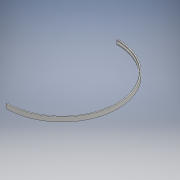
# Autodesk Inventor part: 異形橡膠圈-半圓
Saved by Autodesk Inventor 2018 (Build 220112000, 112)
## iProperties
Created: 2026-01-20
Part Number: 異形橡膠圈-半圓
Material: 一般
Document SubType Name: Modeling
Designer: User
Density: 1 g/cm^3
Appearance: 預設
Author: User
Autodesk Inventor part; units mm, degrees
ref_plane "YZ Plane" through (0, 0, 0) normal (1, 0, 0) x (0, 1, 0)
ref_plane "XZ Plane" through (0, 0, 0) normal (0, 1, 0) x (-1, 0, 0)
ref_plane "XY Plane" through (0, 0, 0) normal (0, 0, 1) x (1, 0, 0)
sketch "草圖1" plane through (0, 0, 0) normal (1, 0, 0) x (0, 1, 0)
  line L0 (-312, 12.65) -> (-317, 12.65)
  line L1 (-317, 12.65) -> (-317, -12.65)
  line L2 (-317, -12.65) -> (-312, -12.65)
  line L3 (-308, -12.65) -> (-308, 12.65) construction
  arc A0 (-310.3276, -7.5781) -> (-310.3276, 7.5781) centre (-321.5, 0) ccw
  line L4 (-310.5, -8.1394) -> (-310.5, -11.15)
  line L5 (-310.5, 8.1394) -> (-310.5, 11.15)
  arc A1 (-310.3276, -7.5781) -> (-310.5, -8.1394) centre (-309.5, -8.1394) ccw
  arc A2 (-310.5, 8.1394) -> (-310.3276, 7.5781) centre (-309.5, 8.1394) ccw
  arc A3 (-312, -12.65) -> (-310.5, -11.15) centre (-312, -11.15) ccw
  arc A4 (-310.5, 11.15) -> (-312, 12.65) centre (-312, 11.15) ccw
  line L6 (0, 0) -> (0, 24.9603) construction
  dimension "d0" = 317
  dimension "d1" = 9
  dimension "d2" = 12.65
  dimension "d3" = 25.3
  dimension "d4" = 27
  dimension "d5" = 0
  dimension "d6" = 2.5
  dimension "d7" = 2.5
  dimension "d8" = 2
  dimension "d9" = 2
  dimension "d10" = 3
  dimension "d11" = 3
  constraints: 14 end point, 10 point on circle, 9 tangent, 5 centre point, 3 vertical, 2 parallel, 1 horizontal, 1 perpendicular
  measures "d0" distance from line of L6.start L1
  measures "d1" distance between parallel lines of L1 L3
  measures "d2" distance from line of L6.start L0
  measures "d3" distance between parallel lines of L0 L2
  measures "d4" diameter of A0
  measures "d5" vertical distance of L6.start A0.centre
  measures "d6" distance between parallel lines of L3 L4
  measures "d7" distance between parallel lines of L3 L5
  measures "d8" diameter of A1
  measures "d9" diameter of A2
  measures "d10" diameter of A3
  measures "d11" diameter of A4
revolve "迴轉1" add sketch "草圖1" angle 180 about axis through (0, 0, 0) along (0, 0, 1)
